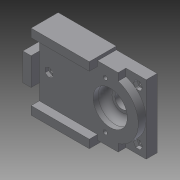
# Autodesk Inventor part: BallBearingCupMountBottom
Saved by Autodesk Inventor 2015 (Build 190159000, 159)
## iProperties
Created: 2017-01-13
Part Number: BallBearingCupMountBottom
Material: Generic
Document SubType Name: Modeling
Designer: 1esh9
Density: 1 g/cm^3
Appearance: Default
Author: 1esh9
Autodesk Inventor part; units mm, degrees
ref_plane "YZ Plane" through (0, 0, 0) normal (1, 0, 0) x (0, 1, 0)
ref_plane "XZ Plane" through (0, 0, 0) normal (0, 1, 0) x (-1, 0, 0)
ref_plane "XY Plane" through (0, 0, 0) normal (0, 0, 1) x (1, 0, 0)
sketch "Sketch1" plane through (0, 0, 0) normal (0, 0, 1) x (1, 0, 0)
  line L0 (0, -8.6) -> (12.34, -8.6) construction
  line L1 (0, 0) -> (0, -8.6)
  line L2 (0, 0) -> (0, -2.1)
  line L3 (0, -2.1) -> (5.3, -2.1)
  line L4 (5.3, -2.1) -> (5.3, 0)
  line L5 (5.3, 0) -> (7.44, 0)
  line L6 (12.44, -8.7) -> (12.44, -5)
  arc A0 (12.44, -5) -> (7.44, 0) centre (7.44, -5) ccw
  line L7 (12.44, -8.7) -> (20.44, -8.7)
  line L8 (20.44, -8.7) -> (20.44, 5)
  line L9 (20.44, 5) -> (0, 5)
  line L10 (0, 5) -> (0, -2.1)
  line L11 (-4.088, 0) -> (24.528, 0) projected
  dimension "d2" = 12.34
  dimension "d3" = 8.6
  dimension "d7" = 0
  dimension "d11" = 5.3
  dimension "d12" = 2.1
  dimension "d14" = 5
  dimension "d15" = 8
  dimension "d16" = 13.7
  dimension "d17" = 3.7
  dimension "d18" = 5
  constraints: 22 end point, 4 perpendicular, 2 collinear, 2 horizontal, 2 point on circle, 2 tangent, 1 centre point, 1 point on line, 1 vertical
  measures "d2" distance of L0.start L0.end
  measures "d3" distance from line of L0 L1.start
  measures "d7" horizontal distance of L1.start L0.start
  measures "d11" distance of L2.end L3.end
  measures "d12" distance of L3.end L4.end
  measures "d14" radius of A0
  measures "d15" distance of L6.start L7.end
  measures "d16" distance of L7.end L8.end
  measures "d17" distance of L6.start L6.end
  measures "d18" distance between parallel lines of L9 L11
revolve "Revolution2" add sketch "Sketch1" angle 360 about axis through (0, 5, 0) along (0, -1, 0)
sketch "Sketch2" plane through (0, 5, 0) normal (0, 1, 0) x (1, 0, 0)
  line L0 (-25, 25) -> (25, 25)
  line L1 (25, 25) -> (25, -25)
  line L2 (25, -25) -> (-25, -25)
  line L3 (-25, -25) -> (-25, 25)
  line L4 (-18.5, 18.5) -> (14.5, 18.5) construction
  line L5 (14.5, 18.5) -> (14.5, -18.5) construction
  line L6 (14.5, -18.5) -> (-18.5, -18.5) construction
  line L7 (-18.5, -18.5) -> (-18.5, 18.5) construction
  circle A0 centre (-18.5, 18.5) radius 1.7
  circle A1 centre (14.5, 18.5) radius 1.7
  circle A2 centre (-18.5, -18.5) radius 1.7
  circle A3 centre (14.5, -18.5) radius 1.7
  line L8 (12.8546, 21.35) -> (16.1454, 21.35)
  line L9 (16.1454, 21.35) -> (17.7909, 18.5)
  line L10 (17.7909, 18.5) -> (16.1454, 15.65)
  line L11 (16.1454, 15.65) -> (12.8546, 15.65)
  line L12 (12.8546, 15.65) -> (11.2091, 18.5)
  line L13 (11.2091, 18.5) -> (12.8546, 21.35)
  line L14 (-17.6058, 15.3329) -> (-20.7956, 16.142)
  line L15 (-20.7956, 16.142) -> (-21.6899, 19.3091)
  line L16 (-21.6899, 19.3091) -> (-19.3942, 21.6671)
  line L17 (-19.3942, 21.6671) -> (-16.2044, 20.858)
  line L18 (-16.2044, 20.858) -> (-15.3101, 17.6909)
  line L19 (-15.3101, 17.6909) -> (-17.6058, 15.3329)
  line L20 (-16.0239, -20.6677) -> (-19.1393, -21.7282)
  line L21 (-19.1393, -21.7282) -> (-21.6153, -19.5605)
  line L22 (-21.6153, -19.5605) -> (-20.9761, -16.3323)
  line L23 (-20.9761, -16.3323) -> (-17.8607, -15.2718)
  line L24 (-17.8607, -15.2718) -> (-15.3847, -17.4395)
  line L25 (-15.3847, -17.4395) -> (-16.0239, -20.6677)
  line L26 (17.7909, -18.5) -> (16.1454, -21.35)
  line L27 (16.1454, -21.35) -> (12.8546, -21.35)
  line L28 (12.8546, -21.35) -> (11.2091, -18.5)
  line L29 (11.2091, -18.5) -> (12.8546, -15.65)
  line L30 (12.8546, -15.65) -> (16.1454, -15.65)
  line L31 (16.1454, -15.65) -> (17.7909, -18.5)
  circle A4 centre (0, 0) radius 12.44 projected
  circle A5 centre (0, 0) radius 12.44 projected
  dimension "d25" = 33
  dimension "d27" = 18.5
  dimension "d28" = 18.5
  dimension "d29" = 37
  dimension "d30" = 3.4
  dimension "d31" = 3.4
  dimension "d32" = 3.4
  dimension "d33" = 3.4
  dimension "d34" = 5.7
  dimension "d36" = 5.7
  dimension "d37" = 5.7
  dimension "d38" = 5.7
  dimension "d39" = 50
  dimension "d40" = 50
  dimension "d41" = 25
  dimension "d42" = 25
  constraints: 64 end point, 8 coincident, 6 parallel, 4 centre point, 2 horizontal, 2 perpendicular, 52 other
  measures "d25" distance of L5.end L6.end
  measures "d27" distance from line of point (0, 0) L7
  measures "d28" distance from line of L4 point (0, 0)
  measures "d29" distance between parallel lines of L4 L6
  measures "d30" diameter of A0
  measures "d31" diameter of A1
  measures "d32" diameter of A2
  measures "d33" diameter of A3
  measures "d34" distance between parallel lines of L27 L30
  measures "d36" distance between parallel lines of L11 L8
  measures "d37" distance between parallel lines of L16 L19
  measures "d38" distance between parallel lines of L22 L25
  measures "d39" distance of L0.start L0.end
  measures "d40" distance of L2.end L0.start
  measures "d41" distance from line of L3 point (0, 0)
  measures "d42" distance from line of point (0, 0) L0
extrude "Extrusion1" add sketch "Sketch2" against normal blind 8 contours L0 L1 L2 L3
extrude "Extrusion2" add sketch "Sketch2" against normal blind 5.5 contours L8 L9 L10 L11 L12 L13 | L14 L15 L16 L17 L18 L19 | L20 L21 L22 L23 L24 L25 | L26 L27 L28 L29 L30 L31
sketch "Sketch4" plane through (0, -2.1, 0) normal (0, -1, 0) x (1, 0, 0)
  circle A0 centre (0, 0) radius 5.3 projected
  point P0 (0, 0)
extrude "Extrusion4" cut sketch "Sketch4" against normal blind 19.5
sketch "Sketch5" plane through (0, -8.7, 0) normal (0, -1, 0) x (1, 0, 0)
  circle A0 centre (0, 0) radius 20.44 projected
  circle A1 centre (0, 0) radius 12.44 projected
  line L0 (-25, -25) -> (25, -25) projected
  line L1 (25, -25) -> (25, 25) projected
  line L2 (25, 25) -> (-25, 25) projected
  line L3 (-25, 25) -> (-25, -25) projected
  line L4 (12.8546, -21.35) -> (11.2091, -18.5) projected
  line L5 (11.2091, -18.5) -> (12.5962, -16.0975) projected
  line L6 (16.1454, -15.65) -> (17.7909, -18.5) projected
  line L7 (17.7909, -18.5) -> (16.1454, -21.35) projected
  line L8 (16.1454, -21.35) -> (12.8546, -21.35) projected
  line L9 (-15.3101, -17.6909) -> (-16.2044, -20.858) projected
  line L10 (-16.2044, -20.858) -> (-19.3942, -21.6671) projected
  line L11 (-19.3942, -21.6671) -> (-21.6899, -19.3091) projected
  line L12 (-21.6899, -19.3091) -> (-20.7956, -16.142) projected
  line L13 (-20.7956, -16.142) -> (-17.6058, -15.3329) projected
  line L14 (-16.0239, 20.6677) -> (-15.3847, 17.4395) projected
  line L15 (-17.8607, 15.2718) -> (-20.9761, 16.3323) projected
  line L16 (-20.9761, 16.3323) -> (-21.6153, 19.5605) projected
  line L17 (-21.6153, 19.5605) -> (-19.1393, 21.7282) projected
  line L18 (-19.1393, 21.7282) -> (-16.0239, 20.6677) projected
  line L19 (17.7909, 18.5) -> (16.1454, 15.65) projected
  line L20 (12.5962, 16.0975) -> (11.2091, 18.5) projected
  line L21 (11.2091, 18.5) -> (12.8546, 21.35) projected
  line L22 (12.8546, 21.35) -> (16.1454, 21.35) projected
  line L23 (16.1454, 21.35) -> (17.7909, 18.5) projected
  arc A2 (12.5962, 16.0975) -> (12.5962, -16.0975) centre (0, 0) ccw projected
  line L24 (-25, 25) -> (3.4372, 20.1489)
  line L25 (-25, -25) -> (3.4372, -20.1489)
  circle A3 centre (0, 0) radius 20.44 projected
  arc A4 (3.4372, 20.1489) -> (3.4372, -20.1489) centre (0, 0) ccw
  line L26 (-25, 25) -> (-51.53, 25)
  line L27 (-51.53, 25) -> (-51.53, -25)
  line L28 (-51.53, -25) -> (-25, -25)
  line L29 (-25, -25) -> (-25, 25)
  line L30 (-17.6058, -15.3329) -> (-15.3101, -17.6909) projected
  line L31 (-15.3847, 17.4395) -> (-17.8607, 15.2718) projected
  arc A5 (13.148, -15.65) -> (13.148, 15.65) centre (0, 0) ccw projected
  line L32 (13.148, -15.65) -> (16.1454, -15.65) projected
  line L33 (16.1454, 15.65) -> (13.148, 15.65) projected
  point P0 (0, 0)
  dimension "d52" = 26.53
  constraints: 12 end point, 4 point on circle, 2 parallel, 2 tangent, 1 centre point, 1 coincident, 1 horizontal, 1 perpendicular, 1 point on line
  measures "d52" distance of L28.end L27.end
extrude "Extrusion5" add sketch "Sketch5" against normal blind 13.7 contours A0 L25 L3 L24 | L3 L28 L27 L26 | L9 L10 L11 L12 L13 L30 | L14 L31 L15 L16 L17 L18
sketch "Sketch6" plane through (-51.53, -8.7, 25) normal (0, -1, 0) x (1, 0, 0)
  arc A0 (54.9672, -45.1489) -> (54.9672, -4.8511) centre (51.53, -25) ccw projected
  line L0 (54.9672, -4.8511) -> (26.53, 0) projected
  line L1 (26.53, 0) -> (0, 0) projected
  line L2 (0, 0) -> (0, -50) projected
  line L3 (0, -50) -> (26.53, -50) projected
  line L4 (26.53, -50) -> (54.9672, -45.1489) projected
  circle A1 centre (51.53, -25) radius 12.44 projected
  line L5 (0, -3.6) -> (42.3, -3.6)
  line L6 (0, -46.4) -> (42.3, -46.4)
  line L7 (9.85, -26.6454) -> (7, -28.2909)
  line L8 (7, -28.2909) -> (4.15, -26.6454)
  line L9 (4.15, -26.6454) -> (4.15, -23.3546)
  line L10 (4.15, -23.3546) -> (7, -21.7091)
  line L11 (7, -21.7091) -> (9.85, -23.3546)
  line L12 (9.85, -23.3546) -> (9.85, -26.6454)
  circle A2 centre (7, -25) radius 1.7
  line L13 (42.3, -3.6) -> (42.3, -2.6902)
  line L14 (42.3, -46.4) -> (42.3, -47.3098)
  point P0 (47.6334, -3.6)
  point P1 (47.6334, -46.4)
  dimension "d55" = 3.6
  dimension "d56" = 3.6
  dimension "d57" = 5.7
  dimension "d58" = 7
  dimension "d59" = 50
  dimension "d60" = 25
  dimension "d61" = 3.4
  dimension "d68" = 42.3
  constraints: 20 end point, 6 point on line, 2 horizontal, 1 centre point, 1 coincident, 1 collinear, 1 parallel, 1 perpendicular, 1 vertical, 13 other
  measures "d55" distance between parallel lines of L1 L5
  measures "d56" distance between parallel lines of L3 L6
  measures "d57" distance between parallel lines of L7 L10
  measures "d58" distance from line of L2 point (7, -25)
  measures "d59" distance of L1.end L2.end
  measures "d60" distance from line of L1 point (7, -25)
  measures "d61" diameter of A2
  measures "d68" distance between parallel lines of L2 L13
extrude "Extrusion6" cut sketch "Sketch6" against normal blind 19.95 contours A2
extrude "Extrusion7" cut sketch "Sketch6" against normal blind 2.5 contours L7 L8 L9 L10 L11 L12
extrude "Extrusion8" add sketch "Sketch6" along normal blind 6 contours L4 L3 L2 L6 L14 | L13 L5 L2 L1 L0
sketch "Sketch7" plane through (0, -8.7, 0) normal (0, -1, 0) x (1, 0, 0)
  line L0 (-9.23, 21.4) -> (-51.53, 21.4) projected
  line L1 (-51.53, 21.4) -> (-51.53, -21.4) projected
  line L2 (-51.53, -21.4) -> (-9.23, -21.4) projected
  line L3 (-9.23, -21.4) -> (-9.23, -22.3098) projected
  line L4 (-9.23, -22.3098) -> (3.4372, -20.1489) projected
  arc A0 (3.4372, -20.1489) -> (3.4372, 20.1489) centre (0, 0) ccw projected
  line L5 (3.4372, 20.1489) -> (-9.23, 22.3098) projected
  line L6 (-9.23, 22.3098) -> (-9.23, 21.4) projected
  line L7 (-41.68, 1.6454) -> (-41.68, -1.6454) projected
  line L8 (-41.68, -1.6454) -> (-44.53, -3.2909) projected
  line L9 (-44.53, -3.2909) -> (-47.38, -1.6454) projected
  line L10 (-47.38, -1.6454) -> (-47.38, 1.6454) projected
  line L11 (-47.38, 1.6454) -> (-44.53, 3.2909) projected
  line L12 (-44.53, 3.2909) -> (-41.68, 1.6454) projected
  circle A1 centre (0, 0) radius 12.44 projected
  line L13 (3.4372, -20.1489) -> (-25, -25) projected
  line L14 (-25, -25) -> (25, -25) projected
  line L15 (25, -25) -> (25, 25) projected
  line L16 (25, 25) -> (-25, 25) projected
  line L17 (-25, 25) -> (3.4372, 20.1489) projected
  arc A2 (3.4372, -20.1489) -> (12.5962, -16.0975) centre (0, 0) ccw projected
  line L18 (12.8546, -21.35) -> (11.2091, -18.5) projected
  line L19 (11.2091, -18.5) -> (12.5962, -16.0975) projected
  line L20 (16.1454, -15.65) -> (17.7909, -18.5) projected
  line L21 (17.7909, -18.5) -> (16.1454, -21.35) projected
  line L22 (16.1454, -21.35) -> (12.8546, -21.35) projected
  line L23 (17.7909, 18.5) -> (16.1454, 15.65) projected
  line L24 (12.5962, 16.0975) -> (11.2091, 18.5) projected
  line L25 (11.2091, 18.5) -> (12.8546, 21.35) projected
  line L26 (12.8546, 21.35) -> (16.1454, 21.35) projected
  line L27 (16.1454, 21.35) -> (17.7909, 18.5) projected
  line L28 (-51.53, -25) -> (25, -25) projected
  line L29 (-9.23, -12.44) -> (5.77, -12.44)
  line L30 (5.77, -12.44) -> (5.77, -25)
  line L31 (5.77, -25) -> (-9.23, -25)
  line L32 (-9.23, -25) -> (-9.23, -12.44)
  line L33 (-9.23, -22.3098) -> (-9.23, -21.4) projected
  line L34 (-9.23, 12.44) -> (5.77, 12.44)
  line L35 (5.77, 12.44) -> (5.77, 25)
  line L36 (5.77, 25) -> (-9.23, 25)
  line L37 (-9.23, 25) -> (-9.23, 12.44)
  line L38 (-9.23, 21.4) -> (-9.23, 22.3098) projected
  circle A3 centre (0, 0) radius 12.44 projected
  line L39 (-9.23, -25) -> (-25, -25)
  line L40 (-25, -25) -> (-9.23, -22.3098)
  line L41 (3.4372, -20.1489) -> (-25, -25) projected
  line L42 (-9.23, -22.3098) -> (-9.23, -25)
  line L43 (-9.23, 22.3098) -> (-9.23, 25)
  line L44 (25, 25) -> (-25, 25) projected
  line L45 (-9.23, 25) -> (-25, 25)
  line L46 (-25, 25) -> (-9.23, 22.3098)
  arc A4 (12.5962, 16.0975) -> (3.4372, 20.1489) centre (0, 0) ccw projected
  line L47 (16.1454, 15.65) -> (13.148, 15.65) projected
  arc A5 (13.148, -15.65) -> (13.148, 15.65) centre (0, 0) ccw projected
  line L48 (13.148, -15.65) -> (16.1454, -15.65) projected
  point P0 (0, 0)
  dimension "d69" = 15
  dimension "d70" = 15
  constraints: 28 end point, 5 collinear, 4 parallel, 4 perpendicular, 3 horizontal, 2 tangent, 1 point on line
  measures "d69" distance between parallel lines of L32 L30
  measures "d70" distance between parallel lines of L37 L35
extrude "Extrusion9" add sketch "Sketch7" against normal blind 6 contours L6 L5 A0 L35 L34 L37 | L37 L16 L35 A0 L5 | L17 L16 L37 | L32 L29 L30 A0 L4 L3 | L32 L14 L13 | L4 A0 L30 L14 L32
sketch "Sketch8" plane through (-51.53, -8.7, -21.4) normal (0, -1, 0) x (1, 0, 0)
  line L0 (39.8818, 0.25) -> (21.4052, 0.25) construction
  line L1 (26.53, -3.6) -> (57.3, -3.6) projected
  circle A0 centre (36.65, 5.9) radius 1.5 construction
  line L2 (42.3, -0.9098) -> (42.3, 0) construction
  circle A1 centre (47.95, 4.25) radius 1.5
  line L3 (30.1874, 42.55) -> (42.031, 42.55) construction
  line L4 (57.3, 46.4) -> (26.53, 46.4) projected
  circle A2 centre (36.65, 36.9) radius 1.5 construction
  circle A3 centre (47.95, 38.55) radius 1.5
  line L5 (42.3, 42.8) -> (42.3, 43.7098) construction
  point P0 (51.53, 21.4)
  dimension "d73" = 3.85
  dimension "d74" = 5.65
  dimension "d75" = 5.65
  dimension "d76" = 3
  dimension "d77" = 3
  dimension "d78" = 5.65
  dimension "d79" = 4
  dimension "d80" = 3.85
  dimension "d81" = 3
  dimension "d82" = 3
  dimension "d83" = 5.65
  dimension "d84" = 4
  dimension "d86" = 5.65
  dimension "d87" = 5.65
  constraints: 4 centre point, 4 end point, 2 horizontal
  measures "d73" distance between parallel lines of L1 L0
  measures "d74" distance from line of L0 A0.centre
  measures "d75" distance from line of L2 A0.centre
  measures "d76" diameter of A0
  measures "d77" diameter of A1
  measures "d78" distance from line of L2 A1.centre
  measures "d79" distance from line of L0 A1.centre
  measures "d80" distance between parallel lines of L4 L3
  measures "d81" diameter of A3
  measures "d82" diameter of A2
  measures "d83" distance from line of L3 A2.centre
  measures "d84" distance from line of L3 A3.centre
  measures "d86" distance from line of A2.centre L5
  measures "d87" distance from line of L5 A3.centre
extrude "Extrusion10" cut sketch "Sketch8" against normal blind 17
sketch "Sketch9" plane through (-51.53, -8.7, -21.4) normal (0, -1, 0) x (1, 0, 0)
  line L0 (0, 42.8) -> (0, 0) projected
  line L1 (0, 31.4) -> (-6, 31.4)
  line L2 (-6, 31.4) -> (-6, 11.4)
  line L3 (-6, 11.4) -> (0, 11.4)
  line L4 (0, 11.4) -> (0, 31.4)
  line L5 (42.3, 42.8) -> (0, 42.8) projected
  line L6 (0, 0) -> (42.3, 0) projected
  point P0 (51.53, 21.4)
  dimension "d94" = 42.8
  dimension "d95" = 20
  dimension "d96" = 11.4
  dimension "d107" = 6
  constraints: 8 end point, 2 parallel, 1 horizontal, 1 perpendicular, 1 point on line
  measures "d94" distance between parallel lines of L5 L6
  measures "d95" distance of L1.end L2.end
  measures "d96" distance between parallel lines of L5 L1
  measures "d107" distance between parallel lines of L0 L2
extrude "Extrusion11" add sketch "Sketch9" against normal blind 13.7
extrude "Extrusion12" add sketch "Sketch9" along normal blind 6
sketch "Sketch10" plane through (-51.53, -14.7, 25) normal (0, -1, 0) x (1, 0, 0)
  line L0 (26.53, 0) -> (0, 0) projected
  line L1 (0, 0) -> (0, -3.6) projected
  line L2 (0, -3.6) -> (42.3, -3.6) projected
  line L3 (42.3, -3.6) -> (42.3, -2.6902) projected
  line L4 (42.3, -2.6902) -> (26.53, 0) projected
  line L5 (0, -50) -> (26.53, -50) projected
  line L6 (26.53, -50) -> (42.3, -47.3098) projected
  line L7 (42.3, -47.3098) -> (42.3, -46.4) projected
  line L8 (42.3, -46.4) -> (0, -46.4) projected
  line L9 (0, -46.4) -> (0, -50) projected
  line L10 (0, -3.6) -> (42.3, -3.6)
  line L11 (42.3, -3.6) -> (42.3, 2.4)
  line L12 (42.3, 2.4) -> (0, 2.4)
  line L13 (0, 2.4) -> (0, -3.6)
  line L14 (0, -46.4) -> (42.3, -46.4)
  line L15 (42.3, -46.4) -> (42.3, -52.4)
  line L16 (42.3, -52.4) -> (0, -52.4)
  line L17 (0, -52.4) -> (0, -46.4)
  line L18 (42.3, -3.6) -> (42.3, -2.6902) projected
  point P0 (51.53, -25)
  dimension "d101" = 6
  dimension "d102" = 6
  constraints: 16 end point, 4 parallel, 2 horizontal, 2 perpendicular, 1 collinear, 1 point on line
  measures "d101" distance between parallel lines of L14 L16
  measures "d102" distance between parallel lines of L10 L12
extrude "Extrusion13" add sketch "Sketch10" against normal blind 19.7
sketch "Sketch11" plane through (0, -3, 0) normal (0, -1, 0) x (1, 0, 0)
  line L0 (5.77, -25) -> (25, -25) projected
  line L1 (25, 25) -> (20.44, 25)
  line L2 (20.44, 25) -> (20.44, -25)
  line L3 (20.44, -25) -> (25, -25)
  line L4 (25, -25) -> (25, 25)
  arc A0 (5.77, -19.6087) -> (5.77, 19.6087) centre (0, 0) ccw projected
  point P0 (0, 0)
  constraints: 8 end point, 2 parallel, 1 horizontal, 1 perpendicular, 1 point on line, 1 tangent
extrude "Extrusion14" cut sketch "Sketch11" against normal blind 19.7
equation "\"d27\" = 0.5 * d29"
equation "\"d28\" = d27"
equation "\"d36\" = d34"
equation "\"d37\" = d34"
equation "\"d38\" = d34"
equation "\"d41\" = 0.5 * d39"
equation "\"d42\" = d41"
equation "\"d60\" = 0.5 * d59"
equation "\"d96\" = -0.5 * d95 + 0.5 * d94"
body "Solid2"
